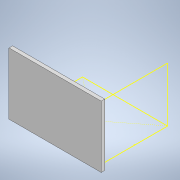
# Autodesk Inventor part: SidePlate
Saved by Autodesk Inventor 2022.2 (Build 262287010, 287A)
## iProperties
Created: 2022-07-12
Part Number: SidePlate
Material: Generic
Document SubType Name: Modeling
Designer: keaton
Density: 1 g/cm^3
Appearance: Default
Author: keaton
Autodesk Inventor part; units mm, degrees
ref_plane "YZ Plane" through (0, 0, 0) normal (1, 0, 0) x (0, 1, 0)
ref_plane "XZ Plane" through (0, 0, 0) normal (0, 1, 0) x (-1, 0, 0)
ref_plane "XY Plane" through (0, 0, 0) normal (0, 0, 1) x (1, 0, 0)
sketch "DeckFace" plane through (0, 0, 0) normal (0, 1, 0) x (-1, 0, 0)
  line L0 (-47.5, 37) -> (47.5, 37)
  line L1 (47.5, 37) -> (47.5, -37)
  line L2 (47.5, -37) -> (-47.5, -37)
  line L3 (-47.5, -37) -> (-47.5, 37)
  line L4 (-47.5, 37) -> (47.5, -37) construction
  line L5 (47.5, 37) -> (-47.5, -37) construction
  point P0 (0, 0)
sketch "DeckSide" plane through (-47.5, 0, 37) normal (0, 0, 1) x (1, 0, 0)
  line L0 (0, 61) -> (95, 61)
  line L1 (0, 0) -> (0, 61)
  line L2 (0, 0) -> (95, 0)
  line L3 (95, 0) -> (95, 61)
  line L4 (99, 65) -> (-4, 65)
  line L5 (-4, 65) -> (-4, -4)
  line L6 (-4, -4) -> (99, -4)
  line L7 (99, -4) -> (99, 65)
  point P0 (47.5, 0)
  dimension "d6" = 4
  measures "d6" distance between parallel lines of L0 L4
sketch "DeckBottom" plane through (47.5, 0, 37) normal (1, 0, 0) x (0, 0, -1)
  line L0 (0, 0) -> (0, 61)
  line L1 (0, 61) -> (74, 61)
  line L2 (74, 0) -> (74, 61)
  line L3 (74, 0) -> (0, 0)
  point P0 (37, 0)
extrude "Extrusion1" add sketch "DeckSide" along normal blind 4 contours L0 L3 L2 L1 | L7 L6 L5 L4
equation "\"d6\" = PlateThickness"
equation "\"d7\" = PlateThickness"
equation "\"PlateThickness\" = 4"
body "Solid1"
